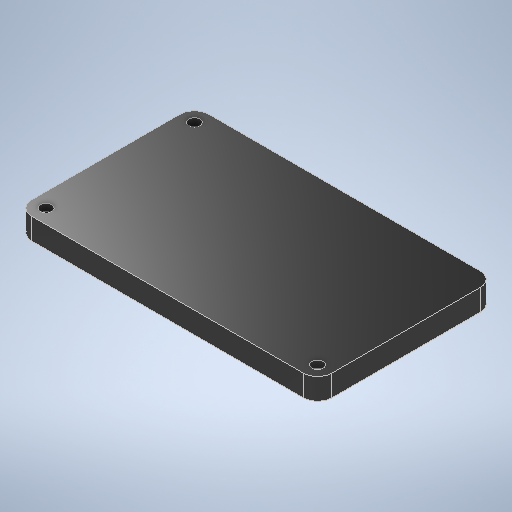
# Autodesk Inventor part: RemoteCasingBackCover
Saved by Autodesk Inventor 2025 (Build 290162000, 162)
## iProperties
Created: 2025-03-09
Part Number: RemoteCasingBackCover
Material: ABS Plastic
Document SubType Name: Modeling
Designer: tvoko
Density: 1.06 g/cm^3
Appearance: Glossy - Black
Author: tvoko
Autodesk Inventor part; units mm, degrees
ref_plane "YZ Plane" through (0, 0, 0) normal (1, 0, 0) x (0, 1, 0)
ref_plane "XZ Plane" through (0, 0, 0) normal (0, 1, 0) x (-1, 0, 0)
ref_plane "XY Plane" through (0, 0, 0) normal (0, 0, 1) x (1, 0, 0)
sketch "Sketch1" plane through (0, 0, 0) normal (0, 1, 0) x (-1, 0, 0)
  line L0 (-2, 0) -> (-78, 0)
  line L1 (-80, -2) -> (-80, -43.5)
  line L2 (-78, -45.5) -> (-2, -45.5)
  line L3 (0, -43.5) -> (0, -2)
  arc A0 (-2, -45.5) -> (0, -43.5) centre (-2, -43.5) ccw
  arc A1 (0, -2) -> (-2, 0) centre (-2, -2) ccw
  arc A2 (-78, 0) -> (-80, -2) centre (-78, -2) ccw
  arc A3 (-80, -43.5) -> (-78, -45.5) centre (-78, -43.5) ccw
  line L4 (2, -2) -> (2, -43.5)
  arc A4 (-2, -47.5) -> (2, -43.5) centre (-2, -43.5) ccw
  line L5 (-2, -47.5) -> (-78, -47.5)
  arc A5 (-82, -43.5) -> (-78, -47.5) centre (-78, -43.5) ccw
  line L6 (-82, -43.5) -> (-82, -2)
  arc A6 (-78, 2) -> (-82, -2) centre (-78, -2) ccw
  line L7 (-78, 2) -> (-2, 2)
  arc A7 (2, -2) -> (-2, 2) centre (-2, -2) ccw
  circle A8 centre (-78, -2) radius 1.6
  circle A9 centre (-2, -43.5) radius 1.6
  circle A10 centre (-2, -2) radius 1.6
  point P0 (0, 0)
  dimension "d0" = 2
  dimension "d1" = 80
  dimension "d3" = 2
  dimension "d9" = 3.2
  dimension "d10" = 45.5
  constraints: 16 end point, 16 point on circle, 11 centre point, 8 tangent, 5 equal radius, 4 parallel, 3 coincident, 2 perpendicular, 2 point on line, 1 horizontal, 7 other
  measures "d0" radius of A0
  measures "d1" distance between parallel lines of L1 L3
  measures "d3" distance between parallel lines of L3 L4
  measures "d9" diameter of A8
  measures "d10" distance between parallel lines of L0 L2
extrude "Extrusion1" add sketch "Sketch1" along normal blind 2 contours A1 L3 A0 L2 A3 L1 A2 L0 | L4 A4 L5 A5 L6 A6 L7 A7
extrude "Extrusion2" add sketch "Sketch1" against normal blind 4 contours L4 A4 L5 A5 L6 A6 L7 A7
body "Solid1"
